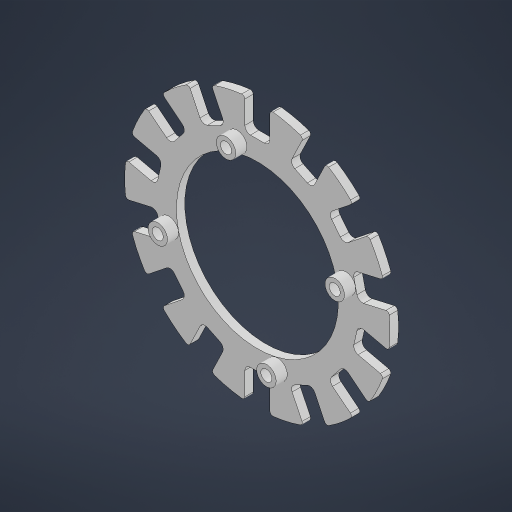
# Autodesk Inventor part: OmniFrame_C
Saved by Autodesk Inventor 2024.2 (Build 282272000, 272)
## iProperties
Created: 2024-02-20
Part Number: OmniFrame_C
Material: 一般
Document SubType Name: Modeling
Designer: Hanaoka
Density: 1 g/cm^3
Appearance: 既定
Author: Hanaoka
Autodesk Inventor part; units mm, degrees
ref_plane "YZ Plane" through (0, 0, 0) normal (1, 0, 0) x (0, 1, 0)
ref_plane "XZ Plane" through (0, 0, 0) normal (0, 1, 0) x (-1, 0, 0)
ref_plane "XY Plane" through (0, 0, 0) normal (0, 0, 1) x (1, 0, 0)
sketch "スケッチ1" plane through (0, 0, 0) normal (0, 0, 1) x (1, 0, 0)
  circle A0 centre (0, 0) radius 25 construction
  line L0 (-2.25, 24.8985) -> (-2.25, 19)
  line L1 (-1.25, 18) -> (1.25, 18)
  line L2 (2.25, 19) -> (2.25, 24.8985)
  line L3 (0, 25) -> (0, 18) construction
  arc A1 (-2.25, 19) -> (-1.25, 18) centre (-1.25, 19) ccw
  arc A2 (1.25, 18) -> (2.25, 19) centre (1.25, 19) ccw
  circle A3 centre (0, 0) radius 23.75
  circle A4 centre (0, 0) radius 17 construction
  line L4 (-3.616, 15.8426) -> (0, 0) construction
  line L5 (0, 0) -> (0, 17) construction
  circle A5 centre (0, 0) radius 14.5
  circle A6 centre (-3.616, 15.8426) radius 1
  circle A7 centre (-3.616, 15.8426) radius 1.75
  circle A8 centre (0, 0) radius 18 construction
  circle A9 centre (-15.8426, -3.616) radius 1.75
  circle A10 centre (-15.8426, -3.616) radius 1
  circle A11 centre (3.616, -15.8426) radius 1.75
  circle A12 centre (3.616, -15.8426) radius 1
  circle A13 centre (15.8426, 3.616) radius 1.75
  circle A14 centre (15.8426, 3.616) radius 1
  line L6 (-12.8303, 21.4566) -> (-10.271, 16.1422)
  line L7 (-6.2166, 18.0946) -> (-8.7759, 23.4091)
  arc A15 (-10.271, 16.1422) -> (-8.9361, 15.6751) centre (-9.37, 16.5761) ccw
  line L8 (-8.9361, 15.6751) -> (-6.6837, 16.7598)
  arc A16 (-6.6837, 16.7598) -> (-6.2166, 18.0946) centre (-7.1176, 17.6608) ccw
  line L9 (-20.8693, 13.7649) -> (-16.2577, 10.0872)
  line L10 (-13.4519, 13.6054) -> (-18.0636, 17.2831)
  arc A17 (-16.2577, 10.0872) -> (-14.8523, 10.2455) centre (-15.6342, 10.869) ccw
  line L11 (-14.8523, 10.2455) -> (-13.2936, 12.2001)
  arc A18 (-13.2936, 12.2001) -> (-13.4519, 13.6054) centre (-14.0754, 12.8236) ccw
  line L12 (-24.775, 3.3469) -> (-19.0243, 2.0343)
  line L13 (-18.023, 6.4215) -> (-23.7736, 7.734)
  arc A19 (-19.0243, 2.0343) -> (-17.8269, 2.7867) centre (-18.8018, 3.0092) ccw
  line L14 (-17.8269, 2.7867) -> (-17.2706, 5.224)
  arc A20 (-17.2706, 5.224) -> (-18.023, 6.4215) centre (-18.2455, 5.4466) ccw
  line L15 (-23.7736, -7.734) -> (-18.023, -6.4215)
  line L16 (-19.0243, -2.0343) -> (-24.775, -3.3469)
  arc A21 (-18.023, -6.4215) -> (-17.2706, -5.224) centre (-18.2455, -5.4466) ccw
  line L17 (-17.2706, -5.224) -> (-17.8269, -2.7867)
  arc A22 (-17.8269, -2.7867) -> (-19.0243, -2.0343) centre (-18.8018, -3.0092) ccw
  line L18 (-18.0636, -17.2831) -> (-13.4519, -13.6054)
  line L19 (-16.2577, -10.0872) -> (-20.8693, -13.7649)
  arc A23 (-13.4519, -13.6054) -> (-13.2936, -12.2001) centre (-14.0754, -12.8236) ccw
  line L20 (-13.2936, -12.2001) -> (-14.8523, -10.2455)
  arc A24 (-14.8523, -10.2455) -> (-16.2577, -10.0872) centre (-15.6342, -10.869) ccw
  line L21 (-8.7759, -23.4091) -> (-6.2166, -18.0946)
  line L22 (-10.271, -16.1422) -> (-12.8303, -21.4566)
  arc A25 (-6.2166, -18.0946) -> (-6.6837, -16.7598) centre (-7.1176, -17.6608) ccw
  line L23 (-6.6837, -16.7598) -> (-8.9361, -15.6751)
  arc A26 (-8.9361, -15.6751) -> (-10.271, -16.1422) centre (-9.37, -16.5761) ccw
  line L24 (2.25, -24.8985) -> (2.25, -19)
  line L25 (-2.25, -19) -> (-2.25, -24.8985)
  arc A27 (2.25, -19) -> (1.25, -18) centre (1.25, -19) ccw
  line L26 (1.25, -18) -> (-1.25, -18)
  arc A28 (-1.25, -18) -> (-2.25, -19) centre (-1.25, -19) ccw
  line L27 (12.8303, -21.4566) -> (10.271, -16.1422)
  line L28 (6.2166, -18.0946) -> (8.7759, -23.4091)
  arc A29 (10.271, -16.1422) -> (8.9361, -15.6751) centre (9.37, -16.5761) ccw
  line L29 (8.9361, -15.6751) -> (6.6837, -16.7598)
  arc A30 (6.6837, -16.7598) -> (6.2166, -18.0946) centre (7.1176, -17.6608) ccw
  line L30 (20.8693, -13.7649) -> (16.2577, -10.0872)
  line L31 (13.4519, -13.6054) -> (18.0636, -17.2831)
  arc A31 (16.2577, -10.0872) -> (14.8523, -10.2455) centre (15.6342, -10.869) ccw
  line L32 (14.8523, -10.2455) -> (13.2936, -12.2001)
  arc A32 (13.2936, -12.2001) -> (13.4519, -13.6054) centre (14.0754, -12.8236) ccw
  line L33 (24.775, -3.3469) -> (19.0243, -2.0343)
  line L34 (18.023, -6.4215) -> (23.7736, -7.734)
  arc A33 (19.0243, -2.0343) -> (17.8269, -2.7867) centre (18.8018, -3.0092) ccw
  line L35 (17.8269, -2.7867) -> (17.2706, -5.224)
  arc A34 (17.2706, -5.224) -> (18.023, -6.4215) centre (18.2455, -5.4466) ccw
  line L36 (23.7736, 7.734) -> (18.023, 6.4215)
  line L37 (19.0243, 2.0343) -> (24.775, 3.3469)
  arc A35 (18.023, 6.4215) -> (17.2706, 5.224) centre (18.2455, 5.4466) ccw
  line L38 (17.2706, 5.224) -> (17.8269, 2.7867)
  arc A36 (17.8269, 2.7867) -> (19.0243, 2.0343) centre (18.8018, 3.0092) ccw
  line L39 (18.0636, 17.2831) -> (13.4519, 13.6054)
  line L40 (16.2577, 10.0872) -> (20.8693, 13.7649)
  arc A37 (13.4519, 13.6054) -> (13.2936, 12.2001) centre (14.0754, 12.8236) ccw
  line L41 (13.2936, 12.2001) -> (14.8523, 10.2455)
  arc A38 (14.8523, 10.2455) -> (16.2577, 10.0872) centre (15.6342, 10.869) ccw
  line L42 (8.7759, 23.4091) -> (6.2166, 18.0946)
  line L43 (10.271, 16.1422) -> (12.8303, 21.4566)
  arc A39 (6.2166, 18.0946) -> (6.6837, 16.7598) centre (7.1176, 17.6608) ccw
  line L44 (6.6837, 16.7598) -> (8.9361, 15.6751)
  arc A40 (8.9361, 15.6751) -> (10.271, 16.1422) centre (9.37, 16.5761) ccw
  point P0 (-2.25, 18)
  point P1 (2.25, 18)
  point P2 (-9.8371, 15.2412)
  point P3 (-5.7827, 17.1937)
  point P4 (-7.8099, 16.2174)
  point P5 (-15.4758, 9.4637)
  point P6 (-12.6701, 12.9819)
  point P7 (-14.073, 11.2228)
  point P8 (-18.0494, 1.8118)
  point P9 (-17.048, 6.199)
  point P10 (-17.5487, 4.0054)
  point P11 (-17.048, -6.199)
  point P12 (-18.0494, -1.8118)
  point P13 (-17.5487, -4.0054)
  point P14 (-12.6701, -12.9819)
  point P15 (-15.4758, -9.4637)
  point P16 (-14.073, -11.2228)
  point P17 (-5.7827, -17.1937)
  point P18 (-9.8371, -15.2412)
  point P19 (-7.8099, -16.2174)
  point P20 (2.25, -18)
  point P21 (-2.25, -18)
  point P22 (0, -18)
  point P23 (9.8371, -15.2412)
  point P24 (5.7827, -17.1937)
  point P25 (7.8099, -16.2174)
  point P26 (15.4758, -9.4637)
  point P27 (12.6701, -12.9819)
  point P28 (14.073, -11.2228)
  point P29 (18.0494, -1.8118)
  point P30 (17.048, -6.199)
  point P31 (17.5487, -4.0054)
  point P32 (17.048, 6.199)
  point P33 (18.0494, 1.8118)
  point P34 (17.5487, 4.0054)
  point P35 (12.6701, 12.9819)
  point P36 (15.4758, 9.4637)
  point P37 (14.073, 11.2228)
  point P38 (5.7827, 17.1937)
  point P39 (9.8371, 15.2412)
  point P40 (7.8099, 16.2174)
  point P41 (-22.5497, -7.4547)
  point P42 (-19.8878, -12.9822)
  point P43 (-17.0821, -16.5004)
  point P44 (-12.2856, -20.3255)
  point P45 (-8.2312, -22.278)
  point P46 (-2.25, -23.6432)
  point P47 (2.25, -23.6432)
  point P48 (8.2312, -22.278)
  point P49 (12.2856, -20.3255)
  point P50 (17.0821, -16.5004)
  point P51 (19.8878, -12.9822)
  point P52 (22.5497, -7.4547)
  point P53 (23.5511, -3.0675)
  point P54 (23.5511, 3.0675)
  point P55 (22.5497, 7.4547)
  point P56 (19.8878, 12.9822)
  point P57 (17.0821, 16.5004)
  point P58 (12.2856, 20.3255)
  point P59 (8.2312, 22.278)
  point P60 (2.25, 23.6432)
  point P61 (-2.25, 23.6432)
  point P62 (-8.2312, 22.278)
  point P63 (-12.2856, 20.3255)
  point P64 (-17.0821, 16.5004)
  point P65 (-19.8878, 12.9822)
  point P66 (-22.5497, 7.4547)
  point P67 (-23.5511, 3.0675)
  point P68 (-23.5511, -3.0675)
  dimension "d13" = 47.5
  dimension "d14" = 34
  dimension "d4" = 50
  dimension "d5" = 4.5
  dimension "d9" = 1
  dimension "d10" = 7
  dimension "d15" = 12.857
  dimension "d16" = 2
  dimension "d17" = 3.5
  dimension "d21" = 360
  dimension "d25" = 360
  constraints: 90 end point, 59 point on circle, 56 point on line, 39 centre point, 13 coincident, 7 tangent, 2 parallel, 2 perpendicular, 2 vertical, 1 equal radius, 1 midpoint, 1 vertical alignment, 246 other
  measures "d4" diameter of A0
  measures "d5" distance of point (-2.25, 18) point (2.25, 18)
  measures "d9" radius of A1
  measures "d10" distance of L3.start L3.end
  measures "d15" angle of L5 L4
  measures "d16" diameter of A6
  measures "d17" diameter of A7
extrude "押し出し1" add sketch "スケッチ1" along normal blind 1.5 contours A7 | L0 A1 L1 A2 L2 A3 L42 A39 L44 A40 L43 L39 A37 L41 A38 L40 L36 A35 L38 A13 A5 A9 L17 A22 L16 L12 A19 L14 A20 L13 L9 A17 L11 A18 L10 L6 A15 L8 A16 L7 | A11 | A3 L33 A33 L35 A34 L34 L30 A31 L32 A32 L31 L27 A29 L29 A30 L28 L24 A27 L26 A28 L25 L21 A25 L23 A26 L22 L18 A23 L20 A24 L19 L15 A21 L17 A9 A5 A13 L38 A36 L37 | A13 | A9
extrude "押し出し2" add sketch "スケッチ1" along normal blind 3.5 contours A7 | A11 | A13 | A9
fillet "フィレット1" radius 0.5 28 edges at (-22.5497, -7.4547, 0.75) (-23.5511, -3.0675, 0.75) (-23.5511, 3.0675, 0.75) (-22.5497, 7.4547, 0.75) (-19.8878, 12.9822, 0.75) (-17.0821, 16.5004, 0.75) (-12.2856, 20.3255, 0.75) (-8.2312, 22.278, 0.75) (-2.25, 23.6432, 0.75) (2.25, 23.6432, 0.75) (8.2312, 22.278, 0.75) (12.2856, 20.3255, 0.75) (17.0821, 16.5004, 0.75) (19.8878, 12.9822, 0.75) (22.5497, 7.4547, 0.75) (23.5511, 3.0675, 0.75) (23.5511, -3.0675, 0.75) (22.5497, -7.4547, 0.75) (19.8878, -12.9822, 0.75) (17.0821, -16.5004, 0.75) (12.2856, -20.3255, 0.75) (8.2312, -22.278, 0.75) (2.25, -23.6432, 0.75) (-2.25, -23.6432, 0.75) (-8.2312, -22.278, 0.75) (-12.2856, -20.3255, 0.75) (-17.0821, -16.5004, 0.75) (-19.8878, -12.9822, 0.75)
